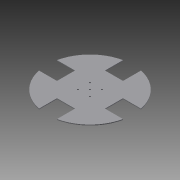
# Autodesk Inventor part: TopCover
Saved by Autodesk Inventor 2013 (Build 170138000, 138)
## iProperties
Created: 2013-08-06
Part Number: TopCover
Material: Generic
Document SubType Name: Sheet Metal
Designer: orange
Density: 1 g/cm^3
Sheet Metal Rule: Default
Author: orange
Autodesk Inventor part; units mm, degrees
ref_plane "YZ Plane" through (0, 0, 0) normal (1, 0, 0) x (0, 1, 0)
ref_plane "XZ Plane" through (0, 0, 0) normal (0, 1, 0) x (-1, 0, 0)
ref_plane "XY Plane" through (0, 0, 0) normal (0, 0, 1) x (1, 0, 0)
sketch "Sketch1" plane through (0, 0, 0) normal (0, 1, 0) x (-1, 0, 0)
  line L0 (38.1, -177.8) -> (38.1, -101.6)
  line L1 (38.1, -101.6) -> (-38.1, -101.6)
  line L2 (-38.1, -101.6) -> (-38.1, -177.8)
  line L3 (38.1, 177.8) -> (38.1, 101.6)
  line L4 (38.1, 101.6) -> (-38.1, 101.6)
  line L5 (-38.1, 101.6) -> (-38.1, 177.8)
  line L6 (177.8, 38.1) -> (101.6, 38.1)
  line L7 (101.6, 38.1) -> (101.6, -38.1)
  line L8 (101.6, -38.1) -> (177.8, -38.1)
  line L9 (-101.6, -38.1) -> (-177.8, -38.1)
  line L10 (-101.6, -38.1) -> (-101.6, 38.1)
  line L11 (-101.6, 38.1) -> (-177.8, 38.1)
  arc A0 (38.1, -177.8) -> (177.8, -38.1) centre (0, 0) ccw
  arc A1 (-177.8, -38.1) -> (-38.1, -177.8) centre (0, 0) ccw
  arc A2 (177.8, 38.1) -> (38.1, 177.8) centre (-0.0019, -0.0019) ccw
  arc A3 (-38.1, 177.8) -> (-177.8, 38.1) centre (0.0019, -0.0019) ccw
  dimension "d0" = 76.2
  dimension "d2" = 76.2
  dimension "d3" = 76.2
  dimension "d4" = 76.2
  dimension "d5" = 76.2
  dimension "d6" = 76.2
  dimension "d7" = 101.6
  dimension "d8" = 101.6
  dimension "d9" = 38.1
  dimension "d10" = 38.1
  dimension "d11" = 76.2
  dimension "d12" = 76.2
  dimension "d13" = 76.2
  dimension "d14" = 101.6
  dimension "d15" = 38.1
  dimension "d16" = 76.2
  dimension "d17" = 76.2
  dimension "d18" = 76.2
  dimension "d19" = 101.6
  dimension "d20" = 38.1
  dimension "d23" = 0
  dimension "d25" = 0
  dimension "d26" = 181.8363
  dimension "d27" = 181.8363
  dimension "d28" = 181.8386
  dimension "d30" = 181.8386
  measures "d0" distance of L0.start L0.end
  measures "d2" distance of L1.end L2.end
  measures "d3" distance of L3.start L3.end
  measures "d4" distance of L4.end L5.end
  measures "d5" distance of L3.end L4.end
  measures "d6" distance of L0.end L1.end
  measures "d7" distance from line of point (0, 0) L1
  measures "d8" distance from line of point (0, 0) L4
  measures "d9" distance from line of point (0, 0) L0
  measures "d10" distance from line of point (0, 0) L3
  measures "d11" distance of L7.end L8.end
  measures "d12" distance of L6.start L6.end
  measures "d13" distance of L6.end L7.end
  measures "d14" distance from line of point (0, 0) L7
  measures "d15" distance from line of point (0, 0) L6
  measures "d16" distance of L9.start L10.end
  measures "d17" distance of L10.end L11.end
  measures "d18" distance of L9.start L9.end
  measures "d19" distance from line of point (0, 0) L10
  measures "d20" distance from line of point (0, 0) L11
  measures "d23" distance of point (0, 0) A1.centre
  measures "d25" distance of point (0, 0) A0.centre
  measures "d26" radius of A0
  measures "d27" radius of A1
  measures "d28" radius of A2
  measures "d30" radius of A3
extrude "Plate1" add sketch "Sketch1" along normal blind 3.175
sketch "Sketch2" plane through (0, 3.175, 0) normal (0, 1, 0) x (1, 0, 0)
  arc A0 (-177.8, -38.1) -> (-38.1, -177.8) centre (0.0019, 0.0019) ccw projected
  arc A1 (38.1, -177.8) -> (177.8, -38.1) centre (-0.0019, 0.0019) ccw projected
  line L0 (-25.4019, -25.3981) -> (25.3981, -25.3981) construction
  line L1 (25.3981, -25.3981) -> (25.3981, 25.4019) construction
  line L2 (25.3981, 25.4019) -> (-25.4019, 25.4019) construction
  line L3 (-25.4019, 25.4019) -> (-25.4019, -25.3981) construction
  dimension "d50" = 50.8
  dimension "d52" = 50.8
  dimension "d53" = 25.4
  dimension "d54" = 25.4
  constraints: 8 end point, 5 coincident, 2 parallel, 1 horizontal, 1 perpendicular
  measures "d50" distance of L1.end L2.end
  measures "d52" distance of L2.end L0.start
  measures "d53" distance from line of L1 A1.centre
  measures "d54" distance from line of A0.centre L2
hole "Hole2" at (-25.4019, 3.175, -25.4019) at (25.3981, 3.175, -25.4019) at (25.3981, 3.175, 25.3981) at (-25.4019, 3.175, 25.3981) direction (0, -1, 0) diameter 6.35 depth 3.175
sketch "Sketch3" plane through (0, 3.175, 0) normal (0, 1, 0) x (1, 0, 0)
  arc A0 (177.8, 38.1) -> (38.1, 177.8) centre (0, 0) ccw projected
  constraints: 1 coincident
hole "Hole3" at (0, 3.175, 0) direction (0, -1, 0) diameter 6.35 depth 3.175 tip angle 118
equation "\"d2\" = d0"
equation "\"d3\" = d0"
equation "\"d4\" = d0"
equation "\"d5\" = d6"
equation "\"d8\" = d7"
equation "\"d9\" = 0.5 * d6"
equation "\"d10\" = 0.5 * d6"
equation "\"d11\" = d0"
equation "\"d12\" = d0"
equation "\"d13\" = d6"
equation "\"d14\" = d7"
equation "\"d15\" = 0.5 * d6"
equation "\"d16\" = d6"
equation "\"d17\" = d0"
equation "\"d18\" = d0"
equation "\"d60\" = Thickness"
equation "\"d67\" = Thickness"
equation "\"d19\" = d7"
equation "\"d20\" = 0.5 * d6"
equation "\"BendRadius\" = Thickness"
equation "\"BendReliefWidth\" = Thickness"
equation "\"BendReliefDepth\" = 0.5 * Thickness"
equation "\"CornerReliefSize\" = 4 * Thickness"
equation "\"MinimumRemnant\" = 2 * Thickness"
equation "\"TransitionRadius\" = BendRadius"
equation "\"JacobiRadiusSize\" = BendRadius"
equation "\"GapSize\" = Thickness"
equation "\"d31\" = BendRadius"
equation "\"Thickness\" = 3.175"
body "Solid1"
